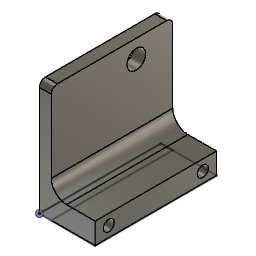
Wrist 1 Side 1 Rev3 (Autodesk Fusion 360 design; units mm, degrees)
Autodesk Fusion 360 part; units mm, degrees
note: some values were not read from the file. Chosen so that the rebuilt part matches the saved one: which face or edge a step refers to. Set by a fixed rule: which sketch regions a step uses.
sketch "Sketch1" plane through (0, 0, 0) normal (0, 0, 1) x (1, 0, 0)
  line L0 (0, 0) -> (18.32, 0)
  line L1 (18.32, 0) -> (18.32, 40)
  line L2 (18.32, 40) -> (0, 40)
  line L3 (0, 40) -> (0, 0)
  line L4 (0, 40) -> (3.9, 40)
  line L5 (3.9, 40) -> (3.9, 0)
  line L6 (3.9, 0) -> (0, 0)
  line L7 (0, 0) -> (0, 40)
  dimension "d1" = 18.32
  dimension "d2" = 40
  dimension "d3" = 3.9
  constraint horizontal L0
  constraint vertical L1
  constraint horizontal L2
  constraint vertical L3
  constraint coincident L0.start L3.end
  constraint horizontal L4
  constraint vertical L5
  constraint horizontal L6
  constraint vertical L7
  measures "d1" distance of L0.start L0.end
  measures "d2" distance of L0.end L1.end
  measures "d3" distance of L2.end L4.end
extrude "Extrude1" add sketch "Sketch1" along normal blind 7 contours L0 L1 L2 L5
extrude "Extrude2" add sketch "Sketch1" along normal blind 38 contours L0 L2 L3 L4 L5 L6 L7
fillet "Fillet1" radius 5 1 edges at (3.9, 20, 7)
sketch "Sketch2" plane through (18.32, 0, 0) normal (1, 0, 0) x (0, 1, 0)
  line L0 (0, 0) -> (40, 0)
  line L1 (40, 0) -> (40, 7)
  line L2 (40, 7) -> (0, 7)
  line L3 (0, 7) -> (0, 0)
  line L4 (0, 3.5) -> (4.5, 3.5)
  line L5 (40, 3.5) -> (35.5, 3.5)
  circle A0 centre (4.5, 3.5) radius 1.8
  circle A1 centre (35.5, 3.5) radius 1.8
  dimension "d9" = 4.5
  dimension "d10" = 4.5
  dimension "d11" = 3.6
  dimension "d12" = 3.6
  constraint midpoint L3 L4.start
  constraint perpendicular L3 L4
  constraint midpoint L1 L5.start
  constraint perpendicular L1 L5
  constraint coincident L4.end A0.centre
  constraint coincident L5.end A1.centre
  measures "d9" distance of L4.start L4.end
  measures "d10" distance of L5.start L5.end
  measures "d11" diameter of A0
  measures "d12" diameter of A1
extrude "Extrude3" cut sketch "Sketch2" against normal up to surface (18.32 mm away) contours A0 | A1
sketch "Sketch3" plane through (0, 0, 0) normal (-1, 0, 0) x (0, -1, 0)
  circle A0 centre (-4.5, 3.5) radius 1.8
  circle A1 centre (-35.5, 3.5) radius 1.8
  line L0 (-40, 0) -> (0, 0)
  line L1 (0, 0) -> (0, 38)
  line L2 (0, 38) -> (-40, 38)
  line L3 (-40, 38) -> (-40, 0)
  line L4 (-40, 38) -> (-28, 38)
  line L5 (-28, 38) -> (-28, 32)
  line L6 (-28, 32) -> (-40, 32)
  line L7 (-40, 32) -> (-40, 38)
  circle A2 centre (-28, 32) radius 3.1
  dimension "d15" = 6.2
  constraint horizontal L4
  constraint vertical L5
  constraint horizontal L6
  constraint vertical L7
  constraint coincident L2.end L3.start
  constraint coincident L5.end L6.start
  measures "d15" diameter of A2
extrude "Extrude4" cut sketch "Sketch3" against normal up to surface (3.9 mm away) contours L5 L6 A2 | L5 L6 A2
fillet "Fillet2" radius 2 1 edges at (1.95, 0, 38)
fillet "Fillet3" radius 2 1 edges at (1.95, 40, 38)
